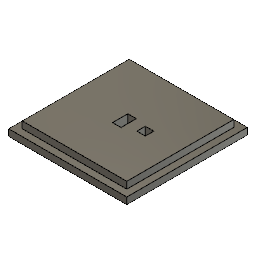
lid version 2 (Autodesk Fusion 360 design; units mm, degrees)
Autodesk Fusion 360 part; units mm, degrees
sketch "Sketch1" plane through (0, 0, 0) normal (0, 1, 0) x (1, 0, 0) in component "Lid"
  line L0 (44.196, 45.085) -> (-44.196, 45.085)
  line L1 (-44.196, 45.085) -> (-44.196, -45.085)
  line L2 (-44.196, -45.085) -> (44.196, -45.085)
  line L3 (44.196, -45.085) -> (44.196, 45.085)
  line L4 (44.196, 45.085) -> (-44.196, -45.085) construction
  line L5 (-44.196, 45.085) -> (44.196, -45.085) construction
  dimension "d1" = 88.392
  dimension "d2" = 90.17
extrude "Extrude1" add sketch "Sketch1" along normal blind 5.08 in component "Lid"
sketch "Sketch3" plane through (0, 5.08, 0) normal (0, 1, 0) x (-1, 0, 0) in component "Lid"
  line L0 (-44.196, 45.085) -> (-44.196, -45.085)
  line L1 (-44.196, -45.085) -> (44.196, -45.085)
  line L2 (44.196, -45.085) -> (44.196, 45.085)
  line L3 (44.196, 45.085) -> (-44.196, 45.085)
  line L4 (-39.116, -40.005) -> (39.116, -40.005)
  line L5 (39.116, -40.005) -> (39.116, 40.005)
  line L6 (39.116, 40.005) -> (-39.116, 40.005)
  line L7 (-39.116, 40.005) -> (-39.116, -40.005)
  line L8 (-39.116, -40.005) -> (39.116, 40.005) construction
  line L9 (39.116, -40.005) -> (-39.116, 40.005) construction
  dimension "d6" = 78.232
  dimension "d7" = 80.01
extrude "Extrude2" add sketch "Sketch3" along normal blind 5.08 contours L4 L5 L6 L7 in component "Lid"
sketch "Sketch6" plane through (0, 0, 0) normal (0, -1, 0) x (1, 0, 0) in component "Lid"
  line L0 (44.196, -45.085) -> (44.196, 45.085)
  line L1 (44.196, 45.085) -> (-44.196, 45.085)
  line L2 (-44.196, 45.085) -> (-44.196, -45.085)
  line L3 (-44.196, -45.085) -> (44.196, -45.085)
  line L4 (2.159, -4.064) -> (-4.191, -4.064)
  line L5 (-4.191, -4.064) -> (-4.191, 7.366)
  line L6 (-4.191, 7.366) -> (2.159, 7.366)
  line L7 (2.159, 7.366) -> (2.159, -4.064)
  line L8 (2.159, -4.064) -> (-4.191, 7.366) construction
  line L9 (-4.191, -4.064) -> (2.159, 7.366) construction
  dimension "d14" = 11.43
  dimension "d15" = 6.35
  dimension "d16" = 1.016
  dimension "d18" = 1.651
  measures "d16" distance of origin
  measures "d18" distance of origin
extrude "Extrude3" cut sketch "Sketch6" against normal blind 10.16 contours L4 L5 L6 L7 in component "Lid"
sketch "Sketch9" plane through (0, 0, 0) normal (0, 1, 0) x (1, 0, 0) in component "Lid"
  line L0 (16.764, -3.81) -> (10.414, -3.81)
  line L1 (10.414, -3.81) -> (10.414, 2.54)
  line L2 (10.414, 2.54) -> (16.764, 2.54)
  line L3 (16.764, 2.54) -> (16.764, -3.81)
  line L4 (16.764, -3.81) -> (10.414, 2.54) construction
  line L5 (10.414, -3.81) -> (16.764, 2.54) construction
  dimension "d28" = 6.35
  dimension "d29" = 6.35
  dimension "d30" = 0.635
  dimension "d31" = 13.589
  measures "d30" distance of origin
  measures "d31" distance of origin
extrude "Extrude5" cut sketch "Sketch9" along normal blind 10.16 in component "Lid"
component "Lid" placed x (1, 0, 0) y (0, 1, 0) z (0, 0, 1) at (0, 0, 0)
